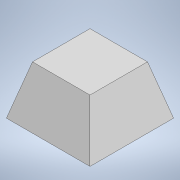
# Autodesk Inventor part: Деталь1
Saved by Autodesk Inventor 2020.1 (Build 241239000, 239)
## iProperties
Created: 2022-03-22
Part Number: Деталь1
Material: Типовые
Document SubType Name: Modeling
Designer: User
Density: 1 g/cm^3
Appearance: По умолчанию
Author: User
Autodesk Inventor part; units mm, degrees
ref_plane "YZ Plane" through (0, 0, 0) normal (1, 0, 0) x (0, 1, 0)
ref_plane "XZ Plane" through (0, 0, 0) normal (0, 1, 0) x (-1, 0, 0)
ref_plane "XY Plane" through (0, 0, 0) normal (0, 0, 1) x (1, 0, 0)
sketch "Эскиз1" plane through (0, 0, 0) normal (0, 0, 1) x (1, 0, 0)
  line L0 (-60, 0) -> (60, 0)
  line L1 (60, 0) -> (41.2436, 70)
  line L2 (41.2436, 70) -> (-41.2436, 70)
  line L3 (-41.2436, 70) -> (-60, 0)
  line L4 (0, 70) -> (0, 0)
  line L5 (-57.3935, 2) -> (-39.7089, 68)
  line L6 (-39.7089, 68) -> (39.7089, 68)
  line L7 (39.7089, 68) -> (57.3935, 2)
  line L8 (57.3935, 2) -> (-57.3935, 2)
  dimension "d0" = 70
  dimension "d1" = 120
  dimension "d2" = 75
  dimension "d8" = 2
  dimension "d9" = 2
  dimension "d10" = 2
  dimension "d11" = 2
  dimension "d12" = 0
  constraints: 18 end point, 4 parallel, 2 horizontal, 1 coincident, 1 midpoint, 1 perpendicular, 1 other
  measures "d0" distance from line of L0 L1.end
  measures "d1" distance of L0.start L0.end
  measures "d2" angle of L1 L0
  measures "d8" distance from line of L0 L7.end
  measures "d9" distance from line of L1 L6.end
  measures "d10" distance from line of L3 L5.end
  measures "d11" distance between parallel lines of L2 L6
  measures "d12" distance from line of L0 L4.end
extrude "Выдавливание1" add sketch "Эскиз1" along normal blind 120 contours L3 L2 L4 L6 L5 L8 L0 | L4 L8 L7 L6 L2 L1 L0
sketch "Эскиз2" plane through (0, 0, 0) normal (1, 0, 0) x (0, 1, 0)
  line L0 (0, 0) -> (0, 120) projected
  line L1 (0, 0) -> (70, 18.7564)
  line L2 (70, 0) -> (70, 120) projected
  line L3 (70, 18.7564) -> (70, 101.2436)
  line L4 (70, 0) -> (70, 120) projected
  line L5 (70, 120) -> (0, 120) projected
  line L6 (70, 101.2436) -> (0, 120)
  line L7 (0, 120) -> (0, 0)
  line L8 (70, 60) -> (0, 60)
  dimension "d5" = 75
  constraints: 10 end point, 2 midpoint, 2 point on line, 1 collinear, 1 perpendicular, 1 other
  measures "d5" angle of L1 L0
extrude "Выдавливание2" cut sketch "Эскиз2" along normal mid plane 1000 contours L0 L8 L2 L1 | L0 L6 L2 L8 keep common part
sketch "Эскиз3" plane through (0, 0, 0) normal (1, 0, 0) x (0, 1, 0)
  line L0 (0, 0) -> (0, 120) projected
  line L1 (70, 18.7564) -> (70, 101.2436) projected
  line L2 (0, 0) -> (70, 18.7564)
  line L3 (70, 18.7564) -> (70, 20.7564)
  line L4 (70, 20.7564) -> (0, 2)
  line L5 (70, 18.7564) -> (0, 0) projected
  line L6 (0, 2) -> (0, 0)
  line L7 (0, 120) -> (70, 101.2436)
  line L8 (68, 101.7795) -> (2, 119.4641) projected
  line L9 (70, 101.2436) -> (70, 99.2436)
  line L10 (70, 99.2436) -> (0, 118)
  line L11 (0, 120) -> (0, 118)
  point P0 (0, 2)
  dimension "d13" = 2
  dimension "d14" = 2
  constraints: 16 end point, 3 parallel, 3 point on line, 2 collinear
  measures "d13" distance of L1.start L3.end
  measures "d14" distance of L1.end L9.end
extrude "Выдавливание3" add sketch "Эскиз3" along normal mid plane 120 contours L0 L4 L1 L2 | L0 L7 L1 L10
sketch "Эскиз4" plane through (0, 0, 0) normal (0, 0, 1) x (1, 0, 0)
  line L0 (60, 70) -> (60, 0) projected
  line L1 (60, 0) -> (41.2436, 70)
  line L2 (60, 70) -> (-60, 70) projected
  line L3 (-41.2436, 70) -> (-60, 0) projected
  line L4 (41.2436, 70) -> (-41.2436, 70)
  line L5 (-41.2436, 70) -> (-60, 0)
  line L6 (-60, 0) -> (60, 0) projected
  line L7 (-60, 0) -> (60, 0)
  line L8 (60, 0) -> (41.2436, 70) projected
  point P0 (0, 0)
  dimension "d19" = 0
  constraints: 8 end point, 2 collinear, 1 horizontal, 1 point on line
  measures "d19" distance from line of L8 L1.end
extrude "Выдавливание4" cut sketch "Эскиз4" along normal blind 120 contours L6 L3 L2 L1 keep common part
